Autodesk Inventor part; units mm, degrees
(part 3 of 3)
  spline S477 degree 2 poles (9.3266, 60.2366) (9.2403, 60.2366) (9.1029, 60.2062) (9.0555, 60.1588) knots 0 0 0 1 2 2 2
  spline S478 degree 2 poles (9.0555, 60.1588) (9.0118, 60.1175) (8.9704, 60.0008) (8.9704, 59.923) knots 0 0 0 1 2 2 2
  line L546 (7.3841, 61) -> (7.6126, 61)
  line L547 (7.6126, 61) -> (7.9773, 60.4019)
  line L548 (7.9773, 60.4019) -> (8.3493, 61)
  line L549 (8.3493, 61) -> (8.5644, 61)
  line L550 (8.5644, 61) -> (8.0867, 60.2488)
  line L551 (8.0867, 60.2488) -> (8.5498, 59.5)
  line L552 (8.5498, 59.5) -> (8.3213, 59.5)
  line L553 (8.3213, 59.5) -> (7.9639, 60.0871)
  line L554 (7.9639, 60.0871) -> (7.5993, 59.5)
  line L555 (7.5993, 59.5) -> (7.3841, 59.5)
  line L556 (7.3841, 59.5) -> (7.8533, 60.2391)
  line L557 (7.8533, 60.2391) -> (7.3841, 61)
  line L558 (6.0908, 60.921) -> (7.1726, 60.4044)
  line L559 (7.1726, 60.4044) -> (7.1726, 60.284)
  line L560 (7.1726, 60.284) -> (6.0908, 59.7674)
  line L561 (6.0908, 59.7674) -> (6.0908, 59.9461)
  line L562 (6.0908, 59.9461) -> (6.9295, 60.3436)
  line L563 (6.9295, 60.3436) -> (6.0908, 60.7423)
  line L564 (6.0908, 60.7423) -> (6.0908, 60.921)
  line L565 (5.2156, 60.4348) -> (5.7832, 60.4348)
  line L566 (5.7832, 60.4348) -> (5.7832, 60.2524)
  line L567 (5.7832, 60.2524) -> (5.2156, 60.2524)
  line L568 (5.2156, 60.2524) -> (5.2156, 60.4348)
  spline S479 degree 2 poles (4.0827, 60.25) (4.0827, 60.6536) (4.3173, 61.0316) (4.5616, 61.0316) knots 0 0 0 1 2 2 2
  spline S480 degree 2 poles (4.5616, 61.0316) (4.8096, 61.0316) (5.0417, 60.6463) (5.0417, 60.2512) knots 0 0 0 1 2 2 2
  spline S481 degree 2 poles (5.0417, 60.2512) (5.0417, 59.8452) (4.8071, 59.4696) (4.5616, 59.4696) knots 0 0 0 1 2 2 2
  spline S482 degree 2 poles (4.5616, 59.4696) (4.3148, 59.4696) (4.0827, 59.8586) (4.0827, 60.25) knots 0 0 0 1 2 2 2
  spline S483 degree 2 poles (4.3404, 60.7071) (4.3112, 60.6329) (4.2869, 60.4044) (4.2869, 60.25) knots 0 0 0 1 2 2 2
  spline S484 degree 2 poles (4.2869, 60.25) (4.2869, 60.0956) (4.3112, 59.8683) (4.3416, 59.7917) knots 0 0 0 1 2 2 2
  spline S485 degree 2 poles (4.3416, 59.7917) (4.372, 59.7152) (4.4777, 59.6361) (4.5616, 59.6361) knots 0 0 0 1 2 2 2
  spline S486 degree 2 poles (4.5616, 59.6361) (4.6455, 59.6361) (4.7536, 59.7152) (4.7853, 59.7942) knots 0 0 0 1 2 2 2
  spline S487 degree 2 poles (4.7853, 59.7942) (4.8156, 59.8707) (4.8375, 60.1041) (4.8375, 60.2512) knots 0 0 0 1 2 2 2
  spline S488 degree 2 poles (4.8375, 60.2512) (4.8375, 60.4092) (4.8181, 60.6207) (4.7865, 60.7034) knots 0 0 0 1 2 2 2
  spline S489 degree 2 poles (4.7865, 60.7034) (4.7573, 60.7812) (4.6491, 60.8651) (4.5616, 60.8651) knots 0 0 0 1 2 2 2
  spline S490 degree 2 poles (4.5616, 60.8651) (4.4789, 60.8651) (4.3707, 60.7861) (4.3404, 60.7071) knots 0 0 0 1 2 2 2
  line L569 (9.2755, 63.5) -> (9.2755, 62.1775)
  line L570 (9.2755, 62.1775) -> (9.7788, 62.1775)
  line L571 (9.7788, 62.1775) -> (9.7788, 62)
  line L572 (9.7788, 62) -> (8.5729, 62)
  line L573 (8.5729, 62) -> (8.5729, 62.1775)
  line L574 (8.5729, 62.1775) -> (9.0762, 62.1775)
  line L575 (9.0762, 62.1775) -> (9.0762, 63.5)
  line L576 (9.0762, 63.5) -> (9.2755, 63.5)
  line L577 (7.3841, 63.5) -> (7.6126, 63.5)
  line L578 (7.6126, 63.5) -> (7.9773, 62.9019)
  line L579 (7.9773, 62.9019) -> (8.3493, 63.5)
  line L580 (8.3493, 63.5) -> (8.5644, 63.5)
  line L581 (8.5644, 63.5) -> (8.0867, 62.7488)
  line L582 (8.0867, 62.7488) -> (8.5498, 62)
  line L583 (8.5498, 62) -> (8.3213, 62)
  line L584 (8.3213, 62) -> (7.9639, 62.5871)
  line L585 (7.9639, 62.5871) -> (7.5993, 62)
  line L586 (7.5993, 62) -> (7.3841, 62)
  line L587 (7.3841, 62) -> (7.8533, 62.7391)
  line L588 (7.8533, 62.7391) -> (7.3841, 63.5)
  line L589 (6.7168, 62.9348) -> (7.2844, 62.9348)
  line L590 (7.2844, 62.9348) -> (7.2844, 62.7524)
  line L591 (7.2844, 62.7524) -> (6.7168, 62.7524)
  line L592 (6.7168, 62.7524) -> (6.7168, 62.9348)
  line L593 (5.3286, 62.9044) -> (6.4105, 63.421)
  line L594 (6.4105, 63.421) -> (6.4105, 63.2423)
  line L595 (6.4105, 63.2423) -> (5.5717, 62.8436)
  line L596 (5.5717, 62.8436) -> (6.4105, 62.4461)
  line L597 (6.4105, 62.4461) -> (6.4105, 62.2674)
  line L598 (6.4105, 62.2674) -> (5.3286, 62.784)
  line L599 (5.3286, 62.784) -> (5.3286, 62.9044)
  line L600 (4.1665, 63.5) -> (4.8983, 63.5)
  line L601 (4.8983, 63.5) -> (4.8983, 63.3468)
  line L602 (4.8983, 63.3468) -> (4.626, 63.3468)
  line L603 (4.626, 63.3468) -> (4.626, 62.3416)
  line L604 (4.626, 62.3416) -> (4.8983, 62.3416)
  line L605 (4.8983, 62.3416) -> (4.8983, 62.2042)
  spline S491 degree 2 poles (4.8983, 62.2042) (4.7439, 62.2042) (4.5981, 62.1167) (4.5883, 61.9951) knots 0 0 0 1 2 2 2
  line L606 (4.5883, 61.9951) -> (4.4327, 61.9951)
  line L607 (4.4327, 61.9951) -> (4.4327, 63.3468)
  line L608 (4.4327, 63.3468) -> (4.1665, 63.3468)
  line L609 (4.1665, 63.3468) -> (4.1665, 63.5)
  point P0 (0, 0)
  dimension "d122" = 0.25
  dimension "d123" = 0.25
  dimension "d124" = 0.25
  dimension "d125" = 0.25
  constraints: 8 collinear, 8 other
  measures "d122" distance between parallel lines of L5 L1
  measures "d123" distance between parallel lines of L12 L9
  measures "d124" distance between parallel lines of L20 L19
  measures "d125" distance between parallel lines of L27 L23
emboss "pinLabels" sketch "pinLabelsSketch" operation add depth 0.0001 direction (0, -1, 0)
ref_plane "Work Plane1" through (0, 9.5, 0) normal (0, 1, 0) x (1, 0, 0)
sketch "Sketch8" plane through (0, 9.5, 0) normal (0, 1, 0) x (1, 0, 0)
  line L0 (49.25, 27) -> (51.75, 27) construction
  line L1 (51.75, 64) -> (49.25, 64) construction
  line L2 (50.5, 64) -> (50.5, 27) construction
  line L3 (1.25, 18.5) -> (3.75, 18.5) construction
  line L4 (3.75, 64) -> (1.25, 64) construction
  line L5 (2.5, 64) -> (2.5, 18.5) construction
  line L6 (49.5, 27.25) -> (49.5, 29.25) construction
  line L7 (49.5, 28.25) -> (51.5, 28.25) construction
  line L8 (51.5, 29.25) -> (51.5, 27.25) construction
  line L9 (49.5, 29.75) -> (49.5, 31.75) construction
  line L10 (49.5, 30.75) -> (51.5, 30.75) construction
  line L11 (51.5, 31.75) -> (51.5, 29.75) construction
  line L12 (49.5, 32.25) -> (49.5, 34.25) construction
  line L13 (49.5, 33.25) -> (51.5, 33.25) construction
  line L14 (51.5, 34.25) -> (51.5, 32.25) construction
  line L15 (49.5, 36.75) -> (49.5, 34.75) construction
  line L16 (49.5, 35.75) -> (51.5, 35.75) construction
  line L17 (51.5, 34.75) -> (51.5, 36.75) construction
  line L18 (49.5, 39.25) -> (49.5, 37.25) construction
  line L19 (49.5, 38.25) -> (51.5, 38.25) construction
  line L20 (51.5, 37.25) -> (51.5, 39.25) construction
  line L21 (49.5, 41.75) -> (49.5, 39.75) construction
  line L22 (49.5, 40.75) -> (51.5, 40.75) construction
  line L23 (51.5, 39.75) -> (51.5, 41.75) construction
  line L24 (51.5, 42.25) -> (51.5, 44.25) construction
  line L25 (51.5, 43.25) -> (49.5, 43.25) construction
  line L26 (49.5, 44.25) -> (49.5, 42.25) construction
  line L27 (51.5, 46.75) -> (51.5, 44.75) construction
  line L28 (51.5, 45.75) -> (49.5, 45.75) construction
  line L29 (49.5, 44.75) -> (49.5, 46.75) construction
  line L30 (51.5, 49.25) -> (51.5, 51.25) construction
  line L31 (51.5, 50.25) -> (49.5, 50.25) construction
  line L32 (49.5, 49.25) -> (49.5, 51.25) construction
  line L33 (51.5, 53.75) -> (51.5, 51.75) construction
  line L34 (51.5, 52.75) -> (49.5, 52.75) construction
  line L35 (49.5, 53.75) -> (49.5, 51.75) construction
  line L36 (51.5, 54.25) -> (51.5, 56.25) construction
  line L37 (51.5, 55.25) -> (49.5, 55.25) construction
  line L38 (49.5, 56.25) -> (49.5, 54.25) construction
  line L39 (49.5, 58.75) -> (49.5, 56.75) construction
  line L40 (49.5, 57.75) -> (51.5, 57.75) construction
  line L41 (51.5, 56.75) -> (51.5, 58.75) construction
  line L42 (49.5, 59.25) -> (49.5, 61.25) construction
  line L43 (49.5, 60.25) -> (51.5, 60.25) construction
  line L44 (51.5, 59.25) -> (51.5, 61.25) construction
  line L45 (49.5, 61.75) -> (49.5, 63.75) construction
  line L46 (49.5, 62.75) -> (51.5, 62.75) construction
  line L47 (51.5, 63.75) -> (51.5, 61.75) construction
  line L48 (1.5, 18.75) -> (1.5, 20.75) construction
  line L49 (1.5, 19.75) -> (3.5, 19.75) construction
  line L50 (3.5, 20.75) -> (3.5, 18.75) construction
  line L51 (3.5, 21.25) -> (3.5, 23.25) construction
  line L52 (3.5, 22.25) -> (1.5, 22.25) construction
  line L53 (1.5, 23.25) -> (1.5, 21.25) construction
  line L54 (1.5, 23.75) -> (1.5, 25.75) construction
  line L55 (1.5, 24.75) -> (3.5, 24.75) construction
  line L56 (3.5, 25.75) -> (3.5, 23.75) construction
  line L57 (1.5, 28.25) -> (1.5, 26.25) construction
  line L58 (1.5, 27.25) -> (3.5, 27.25) construction
  line L59 (3.5, 26.25) -> (3.5, 28.25) construction
  line L60 (1.5, 30.75) -> (1.5, 28.75) construction
  line L61 (1.5, 29.75) -> (3.5, 29.75) construction
  line L62 (1.5, 33.25) -> (1.5, 31.25) construction
  line L63 (1.5, 32.25) -> (3.5, 32.25) construction
  line L64 (3.5, 31.25) -> (3.5, 33.25) construction
  line L65 (3.5, 35.75) -> (3.5, 33.75) construction
  line L66 (3.5, 34.75) -> (1.5, 34.75) construction
  line L67 (1.5, 33.75) -> (1.5, 35.75) construction
  line L68 (3.5, 38.25) -> (3.5, 36.25) construction
  line L69 (3.5, 37.25) -> (1.5, 37.25) construction
  line L70 (1.5, 36.25) -> (1.5, 38.25) construction
  line L71 (3.5, 40.75) -> (3.5, 38.75) construction
  line L72 (3.5, 39.75) -> (1.5, 39.75) construction
  line L73 (1.5, 38.75) -> (1.5, 40.75) construction
  line L74 (1.5, 41.25) -> (1.5, 43.25) construction
  line L75 (1.5, 42.25) -> (3.5, 42.25) construction
  line L76 (3.5, 41.25) -> (3.5, 43.25) construction
  line L77 (1.5, 46.25) -> (1.5, 44.25) construction
  line L78 (1.5, 45.25) -> (3.5, 45.25) construction
  line L79 (3.5, 44.25) -> (3.5, 46.25) construction
  line L80 (3.5, 48.75) -> (3.5, 46.75) construction
  line L81 (3.5, 47.75) -> (1.5, 47.75) construction
  line L82 (1.5, 46.75) -> (1.5, 48.75) construction
  line L83 (3.5, 51.25) -> (3.5, 49.25) construction
  line L84 (3.5, 50.25) -> (1.5, 50.25) construction
  line L85 (1.5, 49.25) -> (1.5, 51.25) construction
  line L86 (1.5, 51.75) -> (1.5, 53.75) construction
  line L87 (1.5, 52.75) -> (3.5, 52.75) construction
  line L88 (3.5, 53.75) -> (3.5, 51.75) construction
  line L89 (3.5, 56.25) -> (3.5, 54.25) construction
  line L90 (3.5, 55.25) -> (1.5, 55.25) construction
  line L91 (1.5, 54.25) -> (1.5, 56.25) construction
  line L92 (3.5, 56.75) -> (3.5, 58.75) construction
  line L93 (3.5, 57.75) -> (1.5, 57.75) construction
  line L94 (1.5, 56.75) -> (1.5, 58.75) construction
  line L95 (1.5, 61.25) -> (1.5, 59.25) construction
  line L96 (1.5, 60.25) -> (3.5, 60.25) construction
  line L97 (3.5, 61.25) -> (3.5, 59.25) construction
  line L98 (3.5, 63.75) -> (3.5, 61.75) construction
  line L99 (3.5, 62.75) -> (1.5, 62.75) construction
  line L100 (1.5, 63.75) -> (1.5, 61.75) construction
  point P0 (0, 0)
  point P1 (50.5, 28.25)
  point P2 (50.5, 30.75)
  point P3 (50.5, 33.25)
  point P4 (50.5, 35.75)
  point P5 (50.5, 38.25)
  point P6 (50.5, 40.75)
  point P7 (50.5, 43.25)
  point P8 (50.5, 45.75)
  point P9 (50.5, 50.25)
  point P10 (50.5, 52.75)
  point P11 (50.5, 55.25)
  point P12 (50.5, 57.75)
  point P13 (50.5, 60.25)
  point P14 (50.5, 62.75)
  point P15 (2.5, 19.75)
  point P16 (2.5, 22.25)
  point P17 (2.5, 24.75)
  point P18 (2.5, 27.25)
  point P19 (2.5, 29.75)
  point P20 (2.5, 32.25)
  point P21 (2.5, 34.75)
  point P22 (2.5, 37.25)
  point P23 (2.5, 39.75)
  point P24 (2.5, 42.25)
  point P25 (2.5, 45.25)
  point P26 (2.5, 47.75)
  point P27 (2.5, 50.25)
  point P28 (2.5, 52.75)
  point P29 (2.5, 55.25)
  point P30 (2.5, 57.75)
  point P31 (2.5, 60.25)
  point P32 (2.5, 62.75)
  constraints: 99 midpoint, 68 end point, 1 horizontal
equation "\"d41\" = d36"
equation "\"d43\" = d38"
equation "\"d44\" = d36"
equation "\"d45\" = d36"
equation "\"d48\" = d38"
